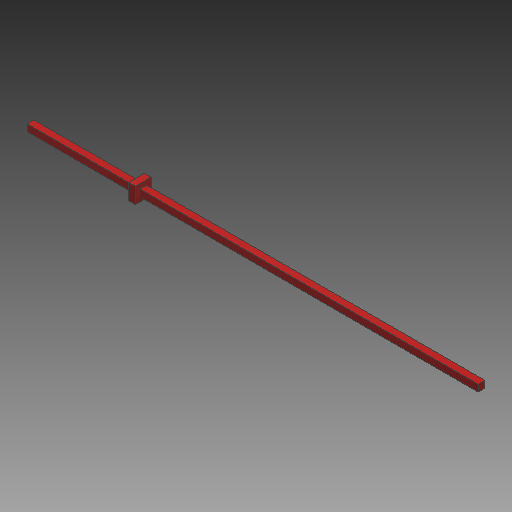
# Autodesk Inventor part: MiddleStick
Saved by Autodesk Inventor 2018.2 (Build 222227000, 227)
## iProperties
Created: 2018-04-10
Part Number: MiddleStick
Material: Generisch
Document SubType Name: Modeling
Designer: Nick Koch
Density: 1 g/cm^3
Appearance: Vorgabe
Author: Nick Koch
Autodesk Inventor part; units mm, degrees
ref_plane "YZ Plane" through (0, 0, 0) normal (1, 0, 0) x (0, 1, 0)
ref_plane "XZ Plane" through (0, 0, 0) normal (0, 1, 0) x (-1, 0, 0)
ref_plane "XY Plane" through (0, 0, 0) normal (0, 0, 1) x (1, 0, 0)
sketch "Skizze4" plane through (0, 0, 0) normal (0, 0, 1) x (1, 0, 0)
  line L0 (0, 0) -> (200, 0)
  line L1 (200, 0) -> (200, 3)
  line L2 (200, 3) -> (0, 3)
  line L3 (0, 3) -> (0, 0)
  dimension "d12" = 200
  dimension "d13" = 3
  constraints: 8 end point, 2 parallel, 1 horizontal, 1 perpendicular
  measures "d12" distance of L2.end L1.end
  measures "d13" distance of L1.end L0.end
extrude "Extrusion4" add sketch "Skizze4" along normal blind 3
sketch "Skizze5" plane through (0, 0, 3) normal (0, 0, 1) x (1, 0, 0)
  line L0 (47, 5) -> (50, 5)
  line L1 (50, 5) -> (50, -2)
  line L2 (50, -2) -> (47, -2)
  line L3 (47, -2) -> (47, 5)
  line L4 (200, 0) -> (200, 3) projected
  line L5 (0, 3) -> (0, 0) projected
  line L6 (200, 3) -> (0, 3) projected
  line L7 (0, 0) -> (200, 0) projected
  dimension "d16" = 150
  dimension "d17" = 47
  dimension "d18" = 2
  dimension "d19" = 2
  constraints: 8 end point, 2 parallel, 1 horizontal, 1 perpendicular
  measures "d16" distance between parallel lines of L4 L1
  measures "d17" distance between parallel lines of L5 L3
  measures "d18" distance between parallel lines of L0 L6
  measures "d19" distance between parallel lines of L7 L2
extrude "Extrusion5" add sketch "Skizze5" along normal blind 2 and the other way blind 5 contours L0 L1 L6 L3 | L6 L1 L7 L3 | L7 L1 L2 L3
